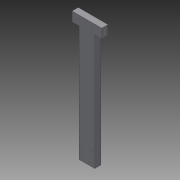
# Autodesk Inventor part: Arm-SquareBar-Rev3
Saved by Autodesk Inventor 2015 (Build 190159000, 159)
## iProperties
Created: 2017-01-08
Part Number: Arm-SquareBar-Rev3
Material: Generic
Document SubType Name: Modeling
Designer: Guy
Density: 1 g/cm^3
Appearance: Default
Mass: 295.484 g
Surface Area: 443.772 cm^2
Volume: 295.484 cm^3
Author: Guy
Autodesk Inventor part; units mm, degrees
ref_plane "YZ Plane" through (0, 0, 0) normal (1, 0, 0) x (0, 1, 0)
ref_plane "XZ Plane" through (0, 0, 0) normal (0, 1, 0) x (-1, 0, 0)
ref_plane "XY Plane" through (0, 0, 0) normal (0, 0, 1) x (1, 0, 0)
sketch "Sketch1" plane through (0, 0, 0) normal (0, 0, 1) x (1, 0, 0)
  line L0 (0, 0) -> (95, 0)
  line L1 (95, 0) -> (95, 20)
  line L2 (95, 20) -> (0, 20)
  line L3 (0, 20) -> (0, 0)
  dimension "d0" = 95
  dimension "d1" = 20
  constraints: 8 end point, 2 parallel, 1 horizontal, 1 perpendicular
  measures "d0" distance of L1.end L2.end
  measures "d1" distance of L0.end L1.end
extrude "Extrusion1" add sketch "Sketch1" along normal blind 400
sketch "Sketch3" plane through (0, 0, 0) normal (-1, 0, 0) x (0, 0, 1)
  line L0 (0, 20) -> (0, 0) projected
  line L1 (0, 0) -> (400, 0) projected
  line L2 (400, 20) -> (400, 0) projected
  line L3 (0, 20) -> (400, 20) projected
  circle A0 centre (390, 10) radius 2.5
  circle A1 centre (380, 10) radius 2.5
  dimension "d18" = 5
  dimension "d19" = 5
  dimension "d22" = 10
  dimension "d24" = 10
  dimension "d26" = 10
  dimension "d27" = 10
  constraints: 2 centre point
  measures "d18" diameter of A0
  measures "d19" diameter of A1
  measures "d22" distance from line of L3 A0.centre
  measures "d24" distance from line of L3 A1.centre
  measures "d26" distance from line of L2 A0.centre
  measures "d27" distance of A1.centre A0.centre
extrude "Extrusion3" cut sketch "Sketch3" against normal through all contours A0 | A1
sketch "Sketch4" plane through (0, 20, 0) normal (0, 1, 0) x (1, 0, 0)
  line L0 (95, 0) -> (0, 0) projected
  line L1 (0, 0) -> (0, -400) projected
  line L2 (95, -400) -> (0, -400) projected
  line L3 (95, 0) -> (95, -400) projected
  line L4 (95, -377.5) -> (95, -382.5) projected
  line L5 (0, -382.5) -> (0, -377.5) projected
  line L6 (95, 0) -> (72.5, 0)
  line L7 (72.5, 0) -> (72.5, -370)
  line L8 (72.5, -370) -> (95, -370)
  line L9 (95, -370) -> (95, 0)
  line L10 (0, 0) -> (22.5, 0)
  line L11 (22.5, 0) -> (22.5, -370)
  line L12 (22.5, -370) -> (0, -370)
  line L13 (0, -370) -> (0, 0)
  dimension "d30" = 30
  dimension "d31" = 50
  dimension "d32" = 22.5
  constraints: 16 end point, 4 parallel, 2 horizontal, 2 perpendicular, 1 point on line
  measures "d30" distance between parallel lines of L12 L2
  measures "d31" distance between parallel lines of L7 L11
  measures "d32" distance between parallel lines of L3 L7
extrude "Extrusion4" cut sketch "Sketch4" against normal up to next contours L3 L8 L7 L0 | L11 L12 L1 L0
sketch "Sketch5" plane through (0, 20, 400) normal (0, 1, 0) x (1, 0, 0)
  circle A0 centre (62.5, 360) radius 2.5
  circle A1 centre (32.5, 360) radius 2.5
  circle A2 centre (62.5, 390) radius 2.5
  circle A3 centre (32.5, 390) radius 2.5
  line L0 (22.5, 400) -> (22.5, 30) projected
  line L1 (22.5, 30) -> (0, 30) projected
  line L2 (0, 30) -> (0, 0) projected
  line L3 (95, 0) -> (0, 0) projected
  line L4 (95, 30) -> (95, 0) projected
  line L5 (95, 30) -> (72.5, 30) projected
  line L6 (72.5, 30) -> (72.5, 400) projected
  line L7 (72.5, 400) -> (22.5, 400) projected
  point P0 (0, 400)
  dimension "d35" = 5
  dimension "d36" = 5
  dimension "d37" = 5
  dimension "d38" = 5
  dimension "d39" = 30
  dimension "d40" = 30
  dimension "d41" = 10
  dimension "d42" = 10
  dimension "d43" = 30
  dimension "d44" = 30
  dimension "d45" = 10
  dimension "d46" = 10
  constraints: 4 centre point
  measures "d35" diameter of A2
  measures "d36" diameter of A3
  measures "d37" diameter of A1
  measures "d38" diameter of A0
  measures "d39" distance of A1.centre A0.centre
  measures "d40" distance of A3.centre A2.centre
  measures "d41" distance from line of L6 A0.centre
  measures "d42" distance from line of L6 A2.centre
  measures "d43" distance of A2.centre A0.centre
  measures "d44" distance of A3.centre A1.centre
  measures "d45" distance from line of L7 A3.centre
  measures "d46" distance from line of L7 A2.centre
extrude "Extrusion5" cut sketch "Sketch5" against normal up to next contours A0 | A1 | A2 | A3
body "Solid1"
